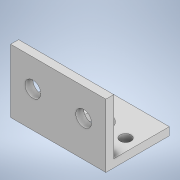
# Autodesk Inventor part: bumper bracket
Saved by Autodesk Inventor 2022 (Build 260153000, 153)
## iProperties
Created: 2023-01-11
Part Number: bumper bracket
Material: Generic
Document SubType Name: Modeling
Designer: s135320
Density: 1 g/cm^3
Appearance: Default
Author: s135320
Autodesk Inventor part; units mm, degrees
ref_plane "YZ Plane" through (0, 0, 0) normal (1, 0, 0) x (0, 1, 0)
ref_plane "XZ Plane" through (0, 0, 0) normal (0, 1, 0) x (-1, 0, 0)
ref_plane "XY Plane" through (0, 0, 0) normal (0, 0, 1) x (1, 0, 0)
sketch "Sketch1" plane through (0, 0, 0) normal (1, 0, 0) x (0, 1, 0)
  line L0 (0, 0) -> (25.4, 0)
  line L1 (25.4, 0) -> (25.4, -25.4)
  line L2 (25.4, -25.4) -> (0, -25.4)
  line L3 (0, -25.4) -> (0, 0)
  line L4 (0, -25.4) -> (3.175, -25.4)
  line L5 (25.4, 0) -> (25.4, -3.175)
  line L6 (25.4, -3.175) -> (3.175, -3.175)
  line L7 (3.175, -3.175) -> (3.175, -25.4)
  dimension "d0" = 25.4
  dimension "d1" = 25.4
  dimension "d2" = 3.175
  dimension "d3" = 3.175
  constraints: 16 end point, 3 perpendicular, 2 parallel, 2 point on line, 1 horizontal
  measures "d0" distance of L1.end L2.end
  measures "d1" distance of L0.end L1.end
  measures "d2" distance of L2.end L4.end
  measures "d3" distance of L0.end L5.end
extrude "Extrusion1" add sketch "Sketch1" along normal blind 38.1 contours L0 L1 L6 L7 L2 L3
sketch "Sketch2" plane through (0, 3.175, -3.175) normal (0, 1, 0) x (1, 0, 0)
  line L0 (0, -3.175) -> (0, 22.225) construction
  line L1 (0, 22.225) -> (0, -3.175) construction
  line L2 (0, 9.525) -> (38.1, 9.525) construction
  line L3 (38.1, -3.175) -> (38.1, 22.225) construction
  circle A0 centre (4.8006, 9.525) radius 2.206
  circle A1 centre (33.2994, 9.525) radius 2.206
  line L4 (33.2994, 9.525) -> (19.05, 9.525) construction
  line L5 (19.05, 9.525) -> (4.8006, 9.525) construction
  line L6 (4.8006, 9.525) -> (22.0472, 9.525) construction
  circle A2 centre (22.0472, 9.525) radius 5.08
  dimension "d6" = 25.4
  dimension "d7" = 14.2494
  dimension "d8" = 14.2494
  dimension "d11" = 4.412
  dimension "d12" = 4.412
  dimension "d15" = 10.16
  dimension "d23" = 11.2522
  constraints: 10 end point, 4 point on line, 3 centre point, 3 midpoint, 1 coincident, 1 collinear, 1 horizontal
  measures "d6" distance of L0.end L1.end
  measures "d7" distance of L4.end L4.start
  measures "d8" distance of L5.end L4.end
  measures "d11" diameter of A1
  measures "d12" diameter of A0
  measures "d15" diameter of A2
  measures "d23" distance of L4.start L6.end
extrude "Extrusion2" cut sketch "Sketch2" against normal blind 38.1
sketch "Sketch3" plane through (0, 3.175, -3.175) normal (0, 0, -1) x (-1, 0, 0)
  line L0 (0, 22.225) -> (0, -3.175) construction
  line L1 (0, 22.225) -> (0, 0) construction
  line L2 (0, 11.1125) -> (-38.1, 11.1125) construction
  line L3 (-38.1, 0) -> (-38.1, 22.225) construction
  circle A0 centre (-29.21, 11.1125) radius 3.175
  circle A1 centre (-8.89, 11.1125) radius 3.175
  line L4 (-19.05, 11.1125) -> (-19.05, 13.4043) construction
  dimension "d16" = 22.225
  dimension "d17" = 10.16
  dimension "d18" = 10.16
  dimension "d19" = 6.35
  dimension "d20" = 6.35
  constraints: 6 end point, 3 midpoint, 3 point on line, 2 centre point, 1 vertical
  measures "d16" distance of L1.end L0.start
  measures "d17" distance of A1.centre L4.start
  measures "d18" distance of A0.centre L4.start
  measures "d19" diameter of A1
  measures "d20" diameter of A0
extrude "Extrusion3" cut sketch "Sketch3" against normal blind 38.1
equation "\"d0\" = d1"
equation "\"d8\" = d7"
equation "\"d12\" = d11"
equation "\"d18\" = d17"
equation "\"d20\" = d19"
body "Solid1"
